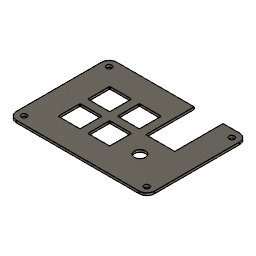
Speedrun pad case top - James - DONE (Autodesk Fusion 360 design; units mm, degrees)
part number: 2026-01-23-14-38-17-234
Autodesk Fusion 360 part; units mm, degrees
sketch "plate-2026-01-23T00_18_16.615Z" plane through (0, 0, 0) normal (0, 0, 1) x (1, 0, 0)
  line L0 (22.075, -21.575) -> (35.075, -21.575)
  line L1 (22.075, -35.575) -> (35.075, -35.575)
  line L2 (21.575, -22.075) -> (21.575, -35.075)
  line L3 (35.575, -22.075) -> (35.575, -35.075)
  arc A0 (22.075, -21.575) -> (21.575, -22.075) centre (22.075, -22.075) ccw
  arc A1 (35.575, -22.075) -> (35.075, -21.575) centre (35.075, -22.075) ccw
  arc A2 (21.575, -35.075) -> (22.075, -35.575) centre (22.075, -35.075) ccw
  arc A3 (35.075, -35.575) -> (35.575, -35.075) centre (35.075, -35.075) ccw
  line L4 (41.125, -21.575) -> (54.125, -21.575)
  line L5 (41.125, -35.575) -> (54.125, -35.575)
  line L6 (40.625, -22.075) -> (40.625, -35.075)
  line L7 (54.625, -22.075) -> (54.625, -35.075)
  arc A4 (41.125, -21.575) -> (40.625, -22.075) centre (41.125, -22.075) ccw
  arc A5 (54.625, -22.075) -> (54.125, -21.575) centre (54.125, -22.075) ccw
  arc A6 (40.625, -35.075) -> (41.125, -35.575) centre (41.125, -35.075) ccw
  arc A7 (54.125, -35.575) -> (54.625, -35.075) centre (54.125, -35.075) ccw
  line L8 (22.075, -40.625) -> (35.075, -40.625)
  line L9 (22.075, -54.625) -> (35.075, -54.625)
  line L10 (21.575, -41.125) -> (21.575, -54.125)
  line L11 (35.575, -41.125) -> (35.575, -54.125)
  arc A8 (22.075, -40.625) -> (21.575, -41.125) centre (22.075, -41.125) ccw
  arc A9 (35.575, -41.125) -> (35.075, -40.625) centre (35.075, -41.125) ccw
  arc A10 (21.575, -54.125) -> (22.075, -54.625) centre (22.075, -54.125) ccw
  arc A11 (35.075, -54.625) -> (35.575, -54.125) centre (35.075, -54.125) ccw
  line L12 (41.125, -40.625) -> (54.125, -40.625)
  line L13 (41.125, -54.625) -> (54.125, -54.625)
  line L14 (40.625, -41.125) -> (40.625, -54.125)
  line L15 (54.625, -41.125) -> (54.625, -54.125)
  arc A12 (41.125, -40.625) -> (40.625, -41.125) centre (41.125, -41.125) ccw
  arc A13 (54.625, -41.125) -> (54.125, -40.625) centre (54.125, -41.125) ccw
  arc A14 (40.625, -54.125) -> (41.125, -54.625) centre (41.125, -54.125) ccw
  arc A15 (54.125, -54.625) -> (54.625, -54.125) centre (54.125, -54.125) ccw
  line L16 (5.423, -5.752) -> (94.148, -5.752)
  line L17 (94.148, -5.752) -> (94.148, -70.327)
  line L18 (94.148, -70.327) -> (5.423, -70.327)
  line L19 (5.423, -70.327) -> (5.423, -5.752)
  line L20 (60.023, -5.752) -> (78.523, -5.752)
  line L21 (78.523, -5.752) -> (78.523, -36.752)
  line L22 (78.523, -36.752) -> (60.023, -36.752)
  line L23 (60.023, -36.752) -> (60.023, -5.752)
  circle A16 centre (10.423, -10.752) radius 1.7
  circle A17 centre (89.148, -10.752) radius 1.7
  circle A18 centre (10.423, -65.327) radius 1.7
  circle A19 centre (89.148, -65.327) radius 1.7
  circle A20 centre (68.898, -49.452) radius 3.5
  dimension "d1" = 64.575
  dimension "d2" = 88.725
  dimension "d3" = 16.152
  dimension "d4" = 15.702
  dimension "d5" = 31
  dimension "d6" = 18.5
  dimension "d7" = 54.6
  dimension "d8" = 3.4
  dimension "d9" = 5
  dimension "d10" = 5
  dimension "d11" = 3.4
  dimension "d12" = 5
  dimension "d13" = 5
  dimension "d14" = 3.4
  dimension "d15" = 5
  dimension "d16" = 5
  dimension "d17" = 3.4
  dimension "d18" = 5
  dimension "d19" = 5
  dimension "d20" = 7
  dimension "d23" = 25.25
  dimension "d24" = 20.875
  constraint horizontal L16
  constraint vertical L17
  constraint horizontal L18
  constraint vertical L19
  constraint horizontal L20
  constraint vertical L21
  constraint horizontal L22
  constraint vertical L23
  constraint coincident L16 L20.start
  measures "d1" distance of L16.start L18.end
  measures "d2" distance of L17 L19
  measures "d3" distance of L10 L19
  measures "d4" distance of L9 L18
  measures "d5" distance of L20.start L22.end
  measures "d6" distance of L21 L23
  measures "d7" distance of L19 L23
  measures "d8" diameter of A16
  measures "d9" distance of L16 A16.centre
  measures "d10" distance of L19 A16.centre
  measures "d11" diameter of A17
  measures "d12" distance of L17 A17.centre
  measures "d13" distance of L16 A17.centre
  measures "d14" diameter of A18
  measures "d15" distance of L19 A18.centre
  measures "d16" distance of L18 A18.centre
  measures "d17" diameter of A19
  measures "d18" distance of L18 A19.centre
  measures "d19" distance of L17 A19.centre
  measures "d20" diameter of A20
  measures "d23" distance of L17 A20.centre
  measures "d24" distance of L18 A20.centre
sketch "Sketch5" plane through (0, 0, 0) normal (0, 0, 1) x (1, 0, 0)
extrude "Extrude1" add sketch "plate-2026-01-23T00_18_16.615Z" along normal blind 1.5 contours L16 L17 L18 L19 L21 L22 L23
fillet "Fillet1" radius 5 4 edges at (94.148, -70.327, 0.75) (94.148, -5.752, 0.75) (5.423, -5.752, 0.75) (5.423, -70.327, 0.75)
sketch "Sketch6" plane through (0, 0, 0) normal (0, 0, -1) x (1, 0, 0)
  circle A0 centre (10.423, 65.327) radius 1.7
  circle A1 centre (68.898, 49.452) radius 3.5
  arc A2 (21.575, 22.075) -> (22.075, 21.575) centre (22.075, 22.075) ccw
  line L0 (21.575, 22.075) -> (21.575, 35.075)
  arc A3 (22.075, 35.575) -> (21.575, 35.075) centre (22.075, 35.075) ccw
  line L1 (22.075, 35.575) -> (35.075, 35.575)
  arc A4 (35.575, 35.075) -> (35.075, 35.575) centre (35.075, 35.075) ccw
  line L2 (35.575, 35.075) -> (35.575, 22.075)
  arc A5 (35.075, 21.575) -> (35.575, 22.075) centre (35.075, 22.075) ccw
  line L3 (35.075, 21.575) -> (22.075, 21.575)
  circle A6 centre (10.423, 10.752) radius 1.7
  arc A7 (40.625, 41.125) -> (41.125, 40.625) centre (41.125, 41.125) ccw
  line L4 (40.625, 41.125) -> (40.625, 54.125)
  arc A8 (41.125, 54.625) -> (40.625, 54.125) centre (41.125, 54.125) ccw
  line L5 (41.125, 54.625) -> (54.125, 54.625)
  arc A9 (54.625, 54.125) -> (54.125, 54.625) centre (54.125, 54.125) ccw
  line L6 (54.625, 54.125) -> (54.625, 41.125)
  arc A10 (54.125, 40.625) -> (54.625, 41.125) centre (54.125, 41.125) ccw
  line L7 (54.125, 40.625) -> (41.125, 40.625)
  circle A11 centre (89.148, 10.752) radius 1.7
  circle A12 centre (89.148, 65.327) radius 1.7
  arc A13 (40.625, 22.075) -> (41.125, 21.575) centre (41.125, 22.075) ccw
  line L8 (40.625, 22.075) -> (40.625, 35.075)
  arc A14 (41.125, 35.575) -> (40.625, 35.075) centre (41.125, 35.075) ccw
  line L9 (41.125, 35.575) -> (54.125, 35.575)
  arc A15 (54.625, 35.075) -> (54.125, 35.575) centre (54.125, 35.075) ccw
  line L10 (54.625, 35.075) -> (54.625, 22.075)
  arc A16 (54.125, 21.575) -> (54.625, 22.075) centre (54.125, 22.075) ccw
  line L11 (54.125, 21.575) -> (41.125, 21.575)
  arc A17 (21.575, 41.125) -> (22.075, 40.625) centre (22.075, 41.125) ccw
  line L12 (21.575, 41.125) -> (21.575, 54.125)
  arc A18 (22.075, 54.625) -> (21.575, 54.125) centre (22.075, 54.125) ccw
  line L13 (22.075, 54.625) -> (35.075, 54.625)
  arc A19 (35.575, 54.125) -> (35.075, 54.625) centre (35.075, 54.125) ccw
  line L14 (35.575, 54.125) -> (35.575, 41.125)
  arc A20 (35.075, 40.625) -> (35.575, 41.125) centre (35.075, 41.125) ccw
  line L15 (35.075, 40.625) -> (22.075, 40.625)
  arc A21 (10.423, 70.327) -> (5.423, 65.327) centre (10.423, 65.327) ccw
  line L16 (5.423, 65.327) -> (5.423, 10.752)
  arc A22 (5.423, 10.752) -> (10.423, 5.752) centre (10.423, 10.752) ccw
  line L17 (10.423, 5.752) -> (60.023, 5.752)
  line L18 (60.023, 5.752) -> (60.023, 36.752)
  line L19 (60.023, 36.752) -> (78.523, 36.752)
  line L20 (78.523, 36.752) -> (78.523, 5.752)
  line L21 (78.523, 5.752) -> (89.148, 5.752)
  arc A23 (89.148, 5.752) -> (94.148, 10.752) centre (89.148, 10.752) ccw
  line L22 (94.148, 10.752) -> (94.148, 65.327)
  arc A24 (94.148, 65.327) -> (89.148, 70.327) centre (89.148, 65.327) ccw
  line L23 (89.148, 70.327) -> (10.423, 70.327)
  line L24 (37.2374, 63.2691) -> (40.5129, 63.2691) construction
  line L25 (40.5129, 63.2691) -> (40.5129, 64.3035) construction
  line L26 (40.5129, 64.3035) -> (37.2374, 64.3035) construction
  line L27 (37.2374, 64.3035) -> (37.2374, 63.2691) construction
  dimension "d29" = 3
  text T0 "Speedrun pad!" font "Arial" height 3 align left top in box 3.2755 x 1.0344 at (37.2374, 63.2691) x (1, 0) y (0, 1) spacing 1
extrude "Extrude2" cut sketch "Sketch6" against normal blind 0.2 text T0
equation "d30 = 'Speedrun pad!'"
